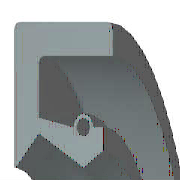
# Autodesk Inventor part: Манжет 2-55x72x8 ГОСТ 8752-79
Saved by Autodesk Inventor 2021 (Build 250183000, 183)
## iProperties
Created: 2020-01-21
Part Number: Манжет 2-55x72x8 ГОСТ 8752-79
Material: Резина
Description: МАНЖЕТЫ РЕЗИНОВЫЕ АРМИРОВАННЫЕ ДЛЯ ВАЛОВ
Document SubType Name: Modeling
Standard: ГОСТ 8752-79-(2)
Designer: gdevc
Standards Organization: GOST
Language: ru-RU
Size Designation: 55 x 72 x 8
Categories: <MemberInstance><Categories><Category DisplayName="Детали вала" InternalName="7f7aeb1f-a693-4053-b835-cee3144e0d98" Mnemonic="SHFT"><Category DisplayName="Уплотнения" InternalName="7cc80d44-b28a-4eb5-95d8-e54d452fb95e" Mnemonic="GSKT"><Category DisplayName="Манжеты" InternalName="b1bc488c-c02d-4af6-ad2b-51fbaea8c3f6" Mnemonic="SLGSKT"><CategoryParameter DisplayName="Диаметр вала" InternalName="0ca11fbe-a678-4712-b689-66c4985a82dc" Mnemonic="shaftdia"/><CategoryParameter DisplayName="Наружный диаметр" InternalName="71be0bee-fd03-42a6-9991-d2da44fa6dc2" Mnemonic="outdia"/><CategoryParameter DisplayName="Толщина" InternalName="c704564b-74bd-4c14-a078-fb73c2ed3f11" Mnemonic="thick"/><CategoryParameter DisplayName="Обозначение размера" InternalName="db3ff616-f16a-4b30-8ba9-6c8f0071faba" Mnemonic="sizedes"/></Category></Category></Category><Category DisplayName="ТипДанных" InternalName="23b78d0f-2648-40c6-8793-ca6db495c9e8" Mnemonic="DATATYPE"><CategoryParameter DisplayName="ОтображаемоеИмя" InternalName="05415f3d-3907-474b-a020-eb9d644f4cf3" Mnemonic="DISPLAYNAME"/><CategoryParameter DisplayName="Стандарт" InternalName="0c0a119c-1e12-4c84-803f-101930972f5e" Mnemonic="STANDARD"/><CategoryParameter DisplayName="Наименование" InternalName="13903e3d-64b1-4950-80da-f627842ea37f" Mnemonic="DESCRIPTION"/><CategoryParameter DisplayName="Обозначение" InternalName="2675968c-4ce5-49e0-a4f5-552d29089031" Mnemonic="DESIGNATION"/><CategoryParameter DisplayName="Строка по умолчанию" InternalName="2af9ec52-faaa-4026-b378-f9fa4afca842" Mnemonic="DEFAULTROW"/><CategoryParameter DisplayName="Имя папки" InternalName="3f06958e-8713-4116-9be7-ed6184ecc97b" Mnemonic="FOLDERNAME"/><CategoryParameter DisplayName="Указатель редакций" InternalName="45a75005-10b1-4dfc-8d6d-dfe629f0b93c" Mnemonic="REVISIONGUID"/><CategoryParameter DisplayName="ИмяФайла" InternalName="8b46a4cc-9585-4fed-90c3-899f57e09a73" Mnemonic="FILENAME"/><CategoryParameter DisplayName="ОргСтанд" InternalName="8f5914e1-4693-403f-8ab5-d37768198c9d" Mnemonic="STDSORG"/><CategoryParameter DisplayName="Версия семейства" InternalName="914462f6-6e19-4b14-ba84-155b9680b1d0" Mnemonic="FAMILYREVISION"/><CategoryParameter DisplayName="Редакция стандарта" InternalName="91d5a463-65c2-4fde-b823-3b7fea5e8e17" Mnemonic="STANDARDREVISION"/><CategoryParameter DisplayName="редакция элемента" InternalName="a65d44b9-392f-4f4f-857b-e4b3d54996fe" Mnemonic="MEMBERREVISION"/><CategoryParameter DisplayName="ФорматКлипа" InternalName="bc51e27b-3422-4e78-93ef-cec197ddf230" Mnemonic="CLIPFORMAT"/><CategoryParameter DisplayName="Изготовитель" InternalName="cd6c7a72-a28a-4e50-99a9-2c7f4e13e5ad" Mnemonic="MANUFACTURER"/><CategoryParameter DisplayName="ВнутреннееИмя" InternalName="cf1d0246-76d9-4b4a-8305-fa0409afb5c1" Mnemonic="INTERNALNAME"/><CategoryParameter DisplayName="Метрическая" InternalName="e2385c5b-1ea4-4823-96a8-8de651266ec3" Mnemonic="ISMETRIC"/><Category DisplayName="Деталь" InternalName="c0e0b642-3bcb-4cc8-9e80-f96d35c4afa4" Mnemonic="PART"><CategoryParameter DisplayName="Номер детали" InternalName="016b6077-bfbe-49bd-92c9-d8d59c39c941" Mnemonic="PARTNUMBER"/><CategoryParameter DisplayName="Инвентарный номер" InternalName="4dba7c1c-e26c-444e-836c-b08b433409a8" Mnemonic="STOCKNUMBER"/><CategoryParameter DisplayName="Ключ материала" InternalName="5c9a8adb-dd2b-4535-b97f-0a94a95fe41f" Mnemonic="MATERIALKEY"/><CategoryParameter DisplayName="Материал" InternalName="818a152a-d3c3-49ca-80ee-df7d91421b8e" Mnemonic="MATERIAL"/></Category></Category><Category DisplayName="СтараяКарта" InternalName="cd87c42b-3e48-431e-b5c0-1cbeb14dfe77" Mnemonic="LEGACYMAP"><CategoryParameter DisplayName="уникальное обозначение элемента DA" InternalName="0918ad47-427f-4fed-ae26-24c81c58f590" Mnemonic="DACOOKIE"/><CategoryParameter DisplayName="Объединить код 11" InternalName="0ee8fb18-e2ed-4f39-96f6-1f4b5f50aa71" Mnemonic="MERGE11"/><CategoryParameter DisplayName="уникальное обозначение элемента CC" InternalName="5193edd4-b2b0-4ab4-9d54-de900eee34e0" Mnemonic="CCCOOKIE"/><CategoryParameter DisplayName="Разделить код" InternalName="72b5c83c-be7f-45c4-ae51-9160ea6deb26" Mnemonic="SPLIT"/><CategoryParameter DisplayName="КодУчастника" InternalName="8e5e0294-fc51-4c8f-b3d7-003dc5ed94f6" Mnemonic="MEMBERID"/><CategoryParameter DisplayName="ИмяКаталога" InternalName="d99d1e27-aa94-4de2-af4c-c348882a6f4f" Mnemonic="CATALOGNAME"/><CategoryParameter DisplayName="НомерСемейства" InternalName="e705e1f4-09cb-413e-91f9-551b4188271e" Mnemonic="FAMILYNUMBER"/></Category></Categories><FamilyTemplate Id="si0061"><FamilyTemplateParameters><FamilyTemplateParameter ObjectType="kUserParameterObject" ValueType="xs:double" Id="1" ObjectReferenceKey="NND"/><FamilyTemplateParameter ObjectType="kUserParameterObject" ValueType="xs:double" Id="2" ObjectReferenceKey="ABDM"/><FamilyTemplateParameter ObjectType="kUserParameterObject" ValueType="xs:double" Id="3" ObjectReferenceKey="RR"/><FamilyTemplateParameter ObjectType="kUserParameterObject" ValueType="xs:double" Id="4" ObjectReferenceKey="LAB"/><FamilyTemplateParameter ObjectType="kUserParameterObject" ValueType="xs:double" Id="5" ObjectReferenceKey="SDI"/><FamilyTemplateParameter ObjectType="kUserParameterObject" ValueType="xs:double" Id="6" ObjectReferenceKey="TKDM"/><FamilyTemplateParameter ObjectType="kUserParameterObject" ValueType="xs:double" Id="7" ObjectReferenceKey="SPDST"/><FamilyTemplateParameter ObjectType="kUserParameterObject" ValueType="xs:double" Id="8" ObjectReferenceKey="SWDT"/><FamilyTemplateParameter ObjectType="kUserParameterObject" ValueType="xs:double" Id="9" ObjectReferenceKey="HLDM"/><FamilyTemplateParameter ObjectType="kUserParameterObject" ValueType="xs:double" Id="10" ObjectReferenceKey="SPDI"/><FamilyTemplateParameter ObjectType="kUserParameterObject" ValueType="xs:double" Id="11" ObjectReferenceKey="SPDA"/><FamilyTemplateParameter ObjectType="kUserParameterObject" ValueType="xs:double" Id="12" ObjectReferenceKey="SD"/><FamilyTemplateParameter ObjectType="kUserParameterObject" ValueType="xs:double" Id="13" ObjectReferenceKey="SD2"/><FamilyTemplateParameter ObjectType="kPropertyObject" ValueType="xs:string" Id="100" ObjectReferenceKey="{32853F0F-3444-11d1-9E93-0060B03C1CA6}" SubObjectId="52"/><FamilyTemplateParameter ObjectType="kPropertyObject" ValueType="xs:string" Id="105" ObjectReferenceKey="{32853F0F-3444-11d1-9E93-0060B03C1CA6}" SubObjectId="5"/><FamilyTemplateParameter ObjectType="kPartComponentDefinitionObject" ValueType="xs:string" Id="110" SubObjectId="Material"/></FamilyTemplateParameters></FamilyTemplate><CategoryParameterMap><ParamToTemplateMap><ParamToTemplate CategoryParameter="//CategoryParameter[@InternalName='05415f3d-3907-474b-a020-eb9d644f4cf3']" ConstantValue="Seal 2 GOST 8752-79"/><ParamToTemplate CategoryParameter="//CategoryParameter[@InternalName='cf1d0246-76d9-4b4a-8305-fa0409afb5c1']" ConstantValue="6ccb1d2b-cd65-4434-9db2-83b487073dc2"/><ParamToTemplate CategoryParameter="//CategoryParameter[@InternalName='3f06958e-8713-4116-9be7-ed6184ecc97b']" ConstantValue="GOST 8752-79(2)"/><ParamToTemplate CategoryParameter="//CategoryParameter[@InternalName='914462f6-6e19-4b14-ba84-155b9680b1d0']" ConstantValue="10"/><ParamToTemplate CategoryParameter="//CategoryParameter[@InternalName='bc51e27b-3422-4e78-93ef-cec197ddf230']" ConstantValue="CF_INVENTOR.STDPARTS"/><ParamToTemplate CategoryParameter="//CategoryParameter[@InternalName='e2385c5b-1ea4-4823-96a8-8de651266ec3']" ConstantValue="true"/><ParamToTemplate CategoryParameter="//CategoryParameter[@InternalName='13903e3d-64b1-4950-80da-f627842ea37f']" ConstantValue="Metal insert rubber seals for rotating shafts"/><ParamToTemplate CategoryParameter="//CategoryParameter[@InternalName='8f5914e1-4693-403f-8ab5-d37768198c9d']" ConstantValue="GOST"/><ParamToTemplate CategoryParameter="//CategoryParameter[@InternalName='0c0a119c-1e12-4c84-803f-101930972f5e']" ConstantValue="GOST 8752-79-(2)"/><ParamToTemplate CategoryParameter="//CategoryParameter[@InternalName='cd6c7a72-a28a-4e50-99a9-2c7f4e13e5ad']" TemplateParameter="104"/><ParamToTemplate CategoryParameter="//CategoryParameter[@InternalName='91d5a463-65c2-4fde-b823-3b7fea5e8e17']" TemplateParameter="103"/><ParamToTemplate CategoryParameter="//CategoryParameter[@InternalName='45a75005-10b1-4dfc-8d6d-dfe629f0b93c']" ConstantValue="5bd53853-20d1-413c-9dc6-47789686271f"/><ParamToTemplate CategoryParameter="//CategoryParameter[@InternalName='2af9ec52-faaa-4026-b378-f9fa4afca842']" ConstantValue="1"/><ParamToTemplate CategoryParameter="//CategoryParameter[@InternalName='d99d1e27-aa94-4de2-af4c-c348882a6f4f']" ConstantValue="GOST"/><ParamToTemplate CategoryParameter="//CategoryParameter[@InternalName='e705e1f4-09cb-413e-91f9-551b4188271e']" ConstantValue="122"/><ParamToTemplate CategoryParameter="//CategoryParameter[@InternalName='8b46a4cc-9585-4fed-90c3-899f57e09a73']" ConstantValue="Манжет 2-55x72x8 ГОСТ 8752-79"/><ParamToTemplate CategoryParameter="//CategoryParameter[@InternalName='a65d44b9-392f-4f4f-857b-e4b3d54996fe']" ConstantValue="b5e1b4b0-e64f-4e25-9682-c464543905a9"/><ParamToTemplate CategoryParameter="//CategoryParameter[@InternalName='db3ff616-f16a-4b30-8ba9-6c8f0071faba']" ConstantValue="55x72x8"/><ParamToTemplate CategoryParameter="//CategoryParameter[@InternalName='8e5e0294-fc51-4c8f-b3d7-003dc5ed94f6']" ConstantValue="49"/><ParamToTemplate CategoryParameter="//CategoryParameter[@InternalName='2675968c-4ce5-49e0-a4f5-552d29089031']" TemplateParameter="100"/><ParamToTemplate CategoryParameter="//CategoryParameter[@InternalName='818a152a-d3c3-49ca-80ee-df7d91421b8e']" TemplateParameter="110"/><ParamToTemplate CategoryParameter="//CategoryParameter[@InternalName='0ca11fbe-a678-4712-b689-66c4985a82dc']" TemplateParameter="1"/><ParamToTemplate CategoryParameter="//CategoryParameter[@InternalName='016b6077-bfbe-49bd-92c9-d8d59c39c941']" TemplateParameter="105"/><ParamToTemplate CategoryParameter="//CategoryParameter[@InternalName='71be0bee-fd03-42a6-9991-d2da44fa6dc2']" TemplateParameter="13"/><ParamToTemplate CategoryParameter="//CategoryParameter[@InternalName='c704564b-74bd-4c14-a078-fb73c2ed3f11']" TemplateParameter="8"/></ParamToTemplateMap></CategoryParameterMap></MemberInstance>
Density: 0.93 g/cm^3
Appearance: Резина — черная
IsCustomPart: 1
Author: gdevc
Autodesk Inventor part; units mm, degrees
ref_plane "YZ Plane" through (0, 0, 0) normal (1, 0, 0) x (0, 1, 0)
ref_plane "XZ Plane" through (0, 0, 0) normal (0, 1, 0) x (-1, 0, 0)
ref_plane "XY Plane" through (0, 0, 0) normal (0, 0, 1) x (1, 0, 0)
sketch "Эскиз1" plane through (0, 0, 0) normal (0, 0, 1) x (1, 0, 0)
  circle A0 centre (5.6, 29.9) radius 0.52
  circle A1 centre (5.6, 29.9) radius 0.8
  line L0 (0, 36) -> (8, 36)
  line L1 (8, 34) -> (2, 34)
  line L2 (0, 0) -> (9.5856, 0)
  line L3 (2, 29.5) -> (5.6, 27.5)
  line L4 (5.6, 27.5) -> (7.2, 28.5)
  line L5 (5.6, 27.5) -> (0, 27.5) construction
  line L6 (0, 18) -> (0, -3) projected
  line L7 (-1.9415, 0) -> (11.5068, 0) projected
  line L8 (4.8, 29.9) -> (2, 30.46)
  line L9 (2, 30.46) -> (2, 34)
  line L10 (0, 36) -> (0, 27.6)
  line L11 (5.6, 27.5) -> (0, 27.5)
  line L12 (2, 29.5) -> (0.1733, 27.532)
  arc A2 (0, 27.6) -> (0.1733, 27.532) centre (0.1, 27.6) ccw
  line L13 (8, 36) -> (8, 34)
  line L14 (6.4, 29.9) -> (7.2, 29.9)
  line L15 (7.2, 29.9) -> (7.2, 28.5)
  point P0 (0, 27.3453)
  dimension "d0" = 72
  dimension "d1" = 2
  dimension "d2" = 1.04
  dimension "d3" = 1.6
  dimension "d4" = 55
  dimension "d5" = 59
  dimension "d7" = 60.92
  dimension "d8" = 2
  dimension "d9" = 5.6
  dimension "d10" = 59.8
  dimension "d11" = 0.1
  dimension "d12" = 7.2
  dimension "d13" = 57
  dimension "d14" = 8
  constraints: 28 end point, 5 horizontal alignment, 5 point on line, 4 point on circle, 4 vertical alignment, 3 centre point, 3 tangent, 2 collinear, 2 horizontal, 2 perpendicular, 1 coincident, 1 parallel
  measures "d0" diameter of L0 L2
  measures "d1" distance of L0.end L1.start
  measures "d2" diameter of A0
  measures "d3" diameter of A1
  measures "d4" diameter of L3.end L2
  measures "d5" diameter of L3.start L2
  measures "d7" diameter of L8.end L2
  measures "d8" distance between parallel lines of L10 L9
  measures "d9" distance from line of L10 A0.centre
  measures "d10" diameter of A0.centre L2
  measures "d11" radius of A2
  measures "d12" distance between parallel lines of L10 L15
  measures "d13" diameter of L4.end L2
  measures "d14" distance from line of L10 L0.end
revolve "Базовый элемент" add sketch "Эскиз1" angle 360 about axis through (0, 0, 0) along (1, 0, 0) contours L14 L15 L4 L3 L12 A2 L10 L0 L13 L1 L9 L8 A1
revolve "Пружинные1" add sketch "Эскиз1" angle 360 about axis through (0, 0, 0) along (1, 0, 0) contours A0 | A1
fillet "Сопряжение1" radius 0.4 3 edges at (8, -36, 0) (2, -34, 0) (0, -36, 0)
equation "\"d0\" = SD2"
equation "\"d1\" = SD"
equation "\"d2\" = SPDI"
equation "\"d3\" = SPDA"
equation "\"d4\" = NND"
equation "\"d5\" = TKDM"
equation "\"d7\" = TKDM + 0.24 * SWDT"
equation "\"d8\" = SD"
equation "\"d9\" = SPDST"
equation "\"d10\" = HLDM"
equation "\"d11\" = 0.25 * LAB"
equation "\"d12\" = SDI"
equation "\"d13\" = ABDM"
equation "\"d14\" = SWDT"
equation "\"d6\" = RR"
equation "\"SD2\" = 72"
equation "\"SWDT\" = 8"
equation "\"RR\" = 0.4"
equation "\"SD\" = 2"
equation "\"NND\" = 55"
equation "\"SPDA\" = 1.6"
equation "\"SPDI\" = 1.04"
equation "\"TKDM\" = 59"
equation "\"HLDM\" = 59.8"
equation "\"ABDM\" = 57"
equation "\"SDI\" = 7.2"
equation "\"SPDST\" = 5.6"
equation "\"LAB\" = 0.4"
body "Solid1"
